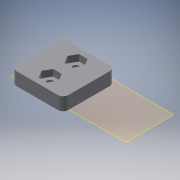
# Autodesk Inventor part: little_holder
Saved by Autodesk Inventor 2016 (Build 200138000, 138)
## iProperties
Created: 2016-01-22
Part Number: little_holder
Material: Generic
Document SubType Name: Modeling
Designer: Erwin Ried
Density: 1 g/cm^3
Appearance: Default
Author: Erwin Ried
Autodesk Inventor part; units mm, degrees
ref_plane "YZ Plane" through (0, 0, 0) normal (1, 0, 0) x (0, 1, 0)
ref_plane "XZ Plane" through (0, 0, 0) normal (0, 1, 0) x (-1, 0, 0)
ref_plane "XY Plane" through (0, 0, 0) normal (0, 0, 1) x (1, 0, 0)
ref_plane "Work Plane1" through (0, 0, 0) normal (0, 0, 1) x (1, 0, 0)
sketch "Sketch1" plane through (0, 0, 0) normal (0, 0, 1) x (1, 0, 0)
  line L0 (7.4216, 7.4531) -> (-20, 7.4531) projected
  line L1 (-20, 7.4531) -> (-20, -9.4531) projected
  line L2 (20, -9.4531) -> (-20, -9.4531) projected
  line L3 (20, -4.1939) -> (20, -9.4531) projected
  line L4 (-20, 7.4531) -> (0, 7.4531)
  line L5 (0, 7.4531) -> (0, -12.5469)
  line L6 (0, -12.5469) -> (-20, -12.5469)
  line L7 (-20, -12.5469) -> (-20, 7.4531)
  arc A0 (8.8358, 6.8673) -> (7.4216, 7.4531) centre (7.4216, 5.4531) ccw projected
  arc A1 (19.5704, -3.8673) -> (20, -4.1939) centre (20.9847, -2.4531) ccw projected
  line L8 (8.8358, 6.8673) -> (19.5704, -3.8673) projected
  point P0 (0, 0)
  dimension "d0" = 20
  dimension "d1" = 20
  constraints: 8 end point, 2 parallel, 1 horizontal, 1 perpendicular
  measures "d0" distance of L5.end L6.end
  measures "d1" distance of L4.end L5.end
extrude "Extrusion1" add sketch "Sketch1" along normal blind 5 contours L5 L2 L1 L0 | L5 L6 L7 L2
fillet "Fillet1" radius 2 4 edges at (0, 7.4531, 2.5) (0, -12.5469, 2.5) (-20, 7.4531, 2.5) (-20, -12.5469, 2.5)
sketch "Sketch2" plane through (0, 0, 5) normal (0, 0, 1) x (1, 0, 0)
  line L0 (-5.26, -4.4531) -> (-16.3573, -5.4531) projected
  arc A0 (-20, -10.5469) -> (-18, -12.5469) centre (-18, -10.5469) ccw projected
  line L1 (-18, -12.5469) -> (-2, -12.5469) projected
  arc A1 (-2, -12.5469) -> (0, -10.5469) centre (-2, -10.5469) ccw projected
  line L2 (0, -10.5469) -> (0, 5.4531) projected
  arc A2 (0, 5.4531) -> (-2, 7.4531) centre (-2, 5.4531) ccw projected
  line L3 (-2, 7.4531) -> (-18, 7.4531) projected
  arc A3 (-18, 7.4531) -> (-20, 5.4531) centre (-18, 5.4531) ccw projected
  line L4 (-20, 5.4531) -> (-20, -10.5469) projected
  line L5 (-10, -12.5469) -> (-10, 7.4531) construction
  line L6 (-2, 7.4531) -> (-18, 7.4531) construction
  line L7 (-10, -2.5469) -> (-10, 2.4531) construction
  line L8 (-10, 2.4531) -> (-10, -7.5469) construction
  point P0 (0, 0)
  dimension "d5" = 5
  dimension "d6" = 10
  constraints: 6 end point, 3 midpoint, 2 point on line
  measures "d5" distance of L7.start L7.end
  measures "d6" distance of L7.end L8.end
hole "Hole1" at (-10, 2.4531, 5) at (-10, -7.5469, 5) direction (0, 0, -1) diameter 3 end through all
sketch "Sketch3" plane through (0, 0, 5) normal (0, 0, 1) x (1, 0, 0)
  circle A0 centre (-10, 2.4531) radius 1.5 projected
  circle A1 centre (-10, -7.5469) radius 1.5 projected
  line L0 (-6.7091, 2.4531) -> (-8.3546, -0.3969)
  line L1 (-8.3546, -0.3969) -> (-11.6454, -0.3969)
  line L2 (-11.6454, -0.3969) -> (-13.2909, 2.4531)
  line L3 (-13.2909, 2.4531) -> (-11.6454, 5.3031)
  line L4 (-11.6454, 5.3031) -> (-8.3546, 5.3031)
  line L5 (-8.3546, 5.3031) -> (-6.7091, 2.4531)
  line L6 (-6.7091, -7.5469) -> (-8.3546, -10.3969)
  line L7 (-8.3546, -10.3969) -> (-11.6454, -10.3969)
  line L8 (-11.6454, -10.3969) -> (-13.2909, -7.5469)
  line L9 (-13.2909, -7.5469) -> (-11.6454, -4.6969)
  line L10 (-11.6454, -4.6969) -> (-8.3546, -4.6969)
  line L11 (-8.3546, -4.6969) -> (-6.7091, -7.5469)
  point P0 (0, 0)
  dimension "d14" = 5.7
  constraints: 24 end point, 2 coincident, 26 other
  measures "d14" distance between parallel lines of L3 L0
extrude "Extrusion2" cut sketch "Sketch3" against normal blind 2.5
body "Solid1"
